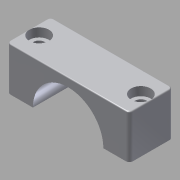
# Autodesk Inventor part: 2.5 CIM mount
Saved by Autodesk Inventor 2013 (Build 170138000, 138)
## iProperties
Created: 2013-01-18
Part Number: 2.5 CIM mount
Material: ABS Plastic
Document SubType Name: Modeling
Designer: Naphat
Density: 1 g/cm^3
Author: Naphat
Autodesk Inventor part; units mm, degrees
ref_plane "YZ Plane" through (0, 0, 0) normal (1, 0, 0) x (0, 1, 0)
ref_plane "XZ Plane" through (0, 0, 0) normal (0, 1, 0) x (-1, 0, 0)
ref_plane "XY Plane" through (0, 0, 0) normal (0, 0, 1) x (1, 0, 0)
sketch "Sketch13" plane through (0, 0, 0) normal (0, 1, 0) x (-1, 0, 0)
  line L0 (0, 0) -> (112, 0)
  line L1 (112, 0) -> (112, 40)
  line L2 (112, 40) -> (0, 40)
  line L3 (0, 40) -> (0, 0)
  dimension "d51" = 112
  dimension "d52" = 40
  constraints: 8 end point, 2 parallel, 1 horizontal, 1 perpendicular
  measures "d51" distance of L2.end L1.end
  measures "d52" distance of L1.end L0.end
extrude "Extrusion11" add sketch "Sketch13" along normal blind 40
sketch "Sketch14" plane through (-112, 0, 40) normal (0, 0, 1) x (1, 0, 0)
  line L0 (0, 0) -> (0, 40) projected
  arc A0 (88.2072, 0) -> (23.7928, 0) centre (56, 0) ccw
  line L1 (23.7928, 0) -> (88.2072, 0)
  dimension "d88" = 32.2072
  constraints: 2 end point, 2 point on circle, 1 centre point, 1 perpendicular
  measures "d88" radius of A0
extrude "Extrusion12" cut sketch "Sketch14" against normal blind 40
sketch "Sketch15" plane through (0, 0, 0) normal (0, -1, 0) x (1, 0, 0)
  line L0 (-88.2072, 0) -> (-88.2072, 40) projected
  line L1 (-112, 40) -> (-88.2072, 40) projected
  line L2 (-112, 0) -> (-112, 40) projected
  line L3 (-88.2072, 0) -> (-112, 0) projected
  line L4 (-100.1315, 0) -> (-100.1315, 2.5) construction
  line L5 (-101.9977, 40) -> (-101.9977, 37.5) construction
  line L6 (-112, 20) -> (-109, 20) construction
  line L7 (-88.2072, 20) -> (-94.2072, 20) construction
  line L8 (-109, 37.5) -> (-96, 37.5)
  line L9 (-96, 37.5) -> (-96, 2.5)
  line L10 (-96, 2.5) -> (-109, 2.5)
  line L11 (-109, 2.5) -> (-109, 37.5)
  line L12 (-23.7928, 40) -> (-23.7928, 0) projected
  line L13 (-23.7928, 40) -> (-23.7928, 0) projected
  line L14 (0, 0) -> (-23.7928, 0) projected
  line L15 (0, 40) -> (0, 0) projected
  line L16 (-23.7928, 40) -> (0, 40) projected
  line L17 (0, 20) -> (-3, 20) construction
  line L18 (-11.8964, 0) -> (-11.8964, 2.5) construction
  line L19 (-11.8964, 40) -> (-11.8964, 37.5) construction
  line L20 (-23.7928, 20) -> (-17.7928, 20) construction
  line L21 (-16, 37.5) -> (-3, 37.5)
  line L22 (-3, 37.5) -> (-3, 2.5)
  line L23 (-3, 2.5) -> (-16, 2.5)
  line L24 (-16, 2.5) -> (-16, 37.5)
  dimension "d60" = 2.5
  dimension "d62" = 2.5
  dimension "d63" = 3
  dimension "d64" = 6
  dimension "d65" = 3
  dimension "d66" = 2.5
  dimension "d67" = 2.5
  dimension "d68" = 6
  constraints: 32 end point, 8 parallel, 6 midpoint, 6 perpendicular, 2 collinear, 2 point on line
  measures "d60" distance of L4.start L4.end
  measures "d62" distance of L5.start L5.end
  measures "d63" distance of L6.start L6.end
  measures "d64" distance of L7.start L7.end
  measures "d65" distance of L17.start L17.end
  measures "d66" distance of L18.start L18.end
  measures "d67" distance of L19.start L19.end
  measures "d68" distance of L20.start L20.end
extrude "Extrusion13" cut sketch "Sketch15" against normal blind 30 contours L8 L9 L10 L11 | L21 L22 L23 L24
sketch "Sketch16" plane through (0, 30, 0) normal (0, -1, 0) x (1, 0, 0)
  line L0 (-16, 37.5) -> (-3, 37.5) projected
  line L1 (-16, 2.5) -> (-16, 37.5) projected
  line L2 (-3, 2.5) -> (-16, 2.5) projected
  line L3 (-3, 37.5) -> (-3, 2.5) projected
  circle A0 centre (-102.5, 20) radius 9
  circle A1 centre (-9.5, 20) radius 9
  point P0 (0, 0)
  dimension "d71" = 18
  dimension "d72" = 18
  constraints: 2 centre point
  measures "d71" diameter of A0
  measures "d72" diameter of A1
extrude "Extrusion14" add sketch "Sketch16" along normal blind 30 contours A1 L3 L1 | L1 A1 | A1 L3 | A0
sketch "Sketch17" plane through (0, 0, 0) normal (0, -1, 0) x (1, 0, 0)
  arc A0 (-109, 13.7751) -> (-96, 13.7751) centre (-102.5, 20) ccw projected
  line L0 (-16, 26.2249) -> (-16, 37.5) projected
  line L1 (-16, 37.5) -> (-3, 37.5) projected
  line L2 (-3, 37.5) -> (-3, 26.2249) projected
  arc A1 (-3, 26.2249) -> (-16, 26.2249) centre (-9.5, 20) ccw projected
  line L3 (-23.7928, 40) -> (-23.7928, 0) projected
  line L4 (0, 0) -> (-23.7928, 0) projected
  line L5 (0, 40) -> (0, 0) projected
  line L6 (-23.7928, 40) -> (0, 40) projected
  arc A2 (-16, 13.7751) -> (-3, 13.7751) centre (-9.5, 20) ccw projected
  line L7 (-3, 13.7751) -> (-3, 2.5) projected
  line L8 (-3, 2.5) -> (-16, 2.5) projected
  line L9 (-16, 2.5) -> (-16, 13.7751) projected
  circle A3 centre (-102.5, 20) radius 5.5
  circle A4 centre (-9.5, 20) radius 5.5
  dimension "d75" = 11
  dimension "d76" = 11
  constraints: 2 centre point, 2 coincident
  measures "d75" diameter of A3
  measures "d76" diameter of A4
extrude "Extrusion15" cut sketch "Sketch17" against normal blind 76.2 contours A3 | A4
sketch "Sketch18" plane through (0, 40, 0) normal (0, 1, 0) x (1, 0, 0)
  circle A0 centre (-102.5, -20) radius 5.5 projected
  circle A1 centre (-9.5, -20) radius 5.5 projected
  circle A2 centre (-102.5, -20) radius 9
  circle A3 centre (-9.5, -20) radius 9
  dimension "d79" = 18
  dimension "d81" = 18
  constraints: 2 centre point, 2 coincident
  measures "d79" diameter of A2
  measures "d81" diameter of A3
extrude "Extrusion16" cut sketch "Sketch18" against normal blind 8
fillet "Fillet3" radius 3.175 6 edges at (-16, 15, 2.5) (-3, 15, 2.5) (-16, 15, 37.5) (-3, 15, 37.5) (0, 20, 40) (0, 20, 0)
fillet "Fillet4" radius 3.175 6 edges at (-112, 20, 0) (-112, 20, 40) (-109, 15, 37.5) (-109, 15, 2.5) (-96, 15, 2.5) (-96, 15, 37.5)
fillet "Fillet5" radius 1 8 edges at (-0.9299, 40, 39.0701) (0, 40, 20) (-0.9299, 40, 0.9299) (-56, 40, 0) (-111.0701, 40, 0.9299) (-112, 40, 20) (-111.0701, 40, 39.0701) (-56, 40, 40)
equation "\"d62\" = d60"
equation "\"d65\" = d63"
equation "\"d66\" = d60"
equation "\"d67\" = d66"
equation "\"d68\" = d64"
equation "\"d81\" = d79"
body "Solid2"
